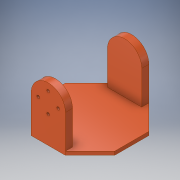
# Autodesk Inventor part: Hipjoint
Saved by Autodesk Inventor 2017 (Build 210142000, 142)
## iProperties
Created: 2017-01-26
Part Number: Hipjoint
Material: PET Plastic
Document SubType Name: Modeling
Designer: Alexander Miller
Density: 1.541 g/cm^3
Appearance: Smooth - Light Orange
Author: Alexander Miller
Autodesk Inventor part; units mm, degrees
ref_plane "YZ Plane" through (0, 0, 0) normal (1, 0, 0) x (0, 1, 0)
ref_plane "XZ Plane" through (0, 0, 0) normal (0, 1, 0) x (-1, 0, 0)
ref_plane "XY Plane" through (0, 0, 0) normal (0, 0, 1) x (1, 0, 0)
sketch "Sketch1" plane through (0, 0, 0) normal (0, 1, 0) x (-1, 0, 0)
  line L0 (-29.25, 29.25) -> (29.25, 29.25)
  line L1 (29.25, 29.25) -> (29.25, -29.25)
  line L2 (29.25, -29.25) -> (-29.25, -29.25)
  line L3 (-29.25, -29.25) -> (-29.25, 29.25)
  point P0 (0, 0)
  point P1 (0, 29.25)
  point P2 (29.25, 0)
  dimension "d0" = 58.5
  dimension "d1" = 58.5
  constraints: 8 end point, 2 midpoint, 2 parallel, 1 horizontal, 1 horizontal alignment, 1 perpendicular, 1 vertical alignment
  measures "d0" distance of L0.start L0.end
  measures "d1" distance of L0.end L1.end
extrude "Extrusion1" add sketch "Sketch1" along normal blind 2.5
sketch "Sketch2" plane through (0, 2.5, 0) normal (0, 1, 0) x (1, 0, 0)
  line L0 (-12, -29.25) -> (12, -29.25)
  line L1 (12, -29.25) -> (12, -24.25)
  line L2 (12, -24.25) -> (-12, -24.25)
  line L3 (-12, -24.25) -> (-12, -29.25)
  line L4 (-40.95, 0) -> (40.95, 0) projected
  line L5 (-12, 29.25) -> (12, 29.25)
  line L6 (12, 29.25) -> (12, 24.25)
  line L7 (12, 24.25) -> (-12, 24.25)
  line L8 (-12, 24.25) -> (-12, 29.25)
  line L9 (-29.25, -29.25) -> (29.25, -29.25) projected
  line L10 (-29.25, 29.25) -> (-29.25, -29.25) projected
  line L11 (29.25, -29.25) -> (29.25, 29.25) projected
  point P0 (0, 0)
  point P1 (0, -24.25)
  dimension "d4" = 5
  dimension "d7" = 24
  constraints: 16 end point, 4 symmetric about line, 2 parallel, 1 collinear, 1 horizontal, 1 midpoint, 1 perpendicular, 1 vertical alignment
  measures "d4" distance between parallel lines of L0 L2
  measures "d7" distance between parallel lines of L1 L3
extrude "Extrusion2" add sketch "Sketch2" along normal blind 35.5 contours L3 L2 L1 L0 | L5 L6 L7 L8
chamfer "Chamfer1" distance 17.25 angle 45 4 edges at (-29.25, 1.25, 29.25) (-29.25, 1.25, -29.25) (29.25, 1.25, -29.25) (29.25, 1.25, 29.25)
full round fillet "Fillet3" first side at (-12, 14.3333, 25.9167) centre faces at (-4, 38, 27.5833) second side at (12, 14.3333, 27.5833)
full round fillet "Fillet4" first side at (-12, 14.3333, -27.5833) centre faces at (-4, 38, -25.9167) second side at (12, 14.3333, -25.9167)
sketch "Sketch3" plane through (-12, 0, 29.25) normal (0, 0, 1) x (1, 0, 0)
  circle A0 centre (12, 26) radius 1.1228 construction
  arc A1 (24, 26) -> (0, 26) centre (12, 26) ccw projected
  circle A2 centre (12, 33) radius 1
  circle A3 centre (5, 26) radius 1
  circle A4 centre (19, 26) radius 1
  circle A5 centre (12, 19) radius 1
  point P0 (12, 0)
  dimension "d13" = 2
  dimension "d14" = 7
  dimension "d15" = 7
  dimension "d16" = 7
  dimension "d17" = 7
  constraints: 5 centre point, 3 equal radius, 2 horizontal alignment, 2 vertical alignment, 1 concentric
  measures "d13" diameter of A2
  measures "d14" distance of A2.centre A0.centre
  measures "d15" distance of A4.centre A0.centre
  measures "d16" distance of A5.centre A0.centre
  measures "d17" distance of A0.centre A3.centre
extrude "Extrusion3" cut sketch "Sketch3" against normal up to surface (5 mm away)
equation "\"d0\" = d1"
equation "\"d1\" = 2.5 * material_thickness + servo_arm_thickness + servo_height + servo_shaft_height"
equation "\"d2\" = 0.5 * material_thickness"
equation "\"d4\" = material_thickness"
equation "\"d7\" = servo_arm_diameter"
equation "\"d5\" = servo_mount_length + servo_arm_diameter + material_thickness"
equation "\"d8\" = -0.5 * servo_arm_diameter + 0.5 * d1"
equation "\"d13\" = servo_arm_hole_diameter"
equation "\"d14\" = servo_arm_hole_distance"
equation "\"d15\" = d14"
equation "\"d16\" = d14"
equation "\"d17\" = d14"
equation "\"material_thickness\" = 5"
equation "\"servo_arm_thickness\" = 2"
equation "\"servo_height\" = 38"
equation "\"servo_shaft_height\" = 6"
equation "\"servo_arm_diameter\" = 24"
equation "\"servo_mount_length\" = 6.5"
equation "\"servo_arm_hole_diameter\" = 2"
equation "\"servo_arm_hole_distance\" = 7"
body "Solid1"
